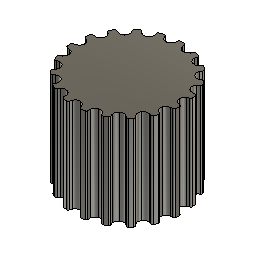
gear_19z (Autodesk Fusion 360 design; units mm, degrees)
Autodesk Fusion 360 part; units mm, degrees
sketch "Sketch1" plane through (0, 0, 0) normal (0, 0, 1) x (1, 0, 0) in component "gt2 pulley"
  circle A0 centre (0, 0) radius 6.0479 construction
  circle A1 centre (0, 0) radius 5.0439 construction
  line L0 (0, 0) -> (0, 6.0479) construction
  line L1 (0, 0) -> (0.9954, 5.9654) construction
  line L2 (0, 0) -> (1.4117, 5.8808) construction
  circle A2 centre (0, 0) radius 5.7939 construction
  arc A3 (0.3524, 5.6394) -> (0.3842, 5.3837) centre (1.3524, 5.6338) ccw
  circle A4 centre (0, 0) radius 5.6439 construction
  arc A5 (0.2077, 5.7902) -> (0, 5.7939) centre (0, 0) ccw
  arc A6 (0.3524, 5.6394) -> (0.2077, 5.7902) centre (0.2024, 5.6403) ccw
  arc A7 (0.3842, 5.3837) -> (0.8302, 4.9751) centre (0.9215, 5.5225) ccw
  arc A8 (0, 5.7939) -> (-0.2077, 5.7902) centre (0, 0) ccw
  arc A9 (-0.2077, 5.7902) -> (-0.3524, 5.6394) centre (-0.2024, 5.6403) ccw
  arc A10 (-0.3842, 5.3837) -> (-0.3524, 5.6394) centre (-1.3524, 5.6338) ccw
  arc A11 (-0.8302, 4.9751) -> (-0.3842, 5.3837) centre (-0.9215, 5.5225) ccw
  arc A12 (0.8302, 4.9751) -> (-0.8302, 4.9751) centre (0, 0) ccw
  point P0 (1.3524, 5.6338)
  point P1 (0, 5.7939)
  dimension "d18" = 12.0958
  dimension "d19" = 9.474
  dimension "d22" = 1.004
  dimension "d24" = 0.75
  dimension "d26" = 1
  dimension "d27" = 0.15
  dimension "d28" = 0.15
  dimension "d47" = 0.555
  dimension "d52" = 3.812
  constraint coincident A0.centre A1.centre
  constraint coincident A0 L0.end
  constraint vertical L0
  constraint coincident A0 L1.end
  constraint coincident A0 L2.end
  constraint concentric A1 A2
  constraint coincident A1 A7.end
  constraint coincident L1 A7.end
  constraint coincident A2 P0
  constraint coincident L2 P0
  constraint coincident P0 A3.centre
  constraint coincident A2 P1
  constraint coincident L0 P1
  constraint concentric A2 A4
  constraint coincident P1 A5.end
  constraint coincident A4 A6.centre
  constraint coincident A3.start A6.start
  constraint tangent A3 A6
  constraint tangent A3 A7
  constraint symmetric L0 A7.end A11.start
  constraint symmetric L0 A3.start A9.end
  constraint symmetric L0 A3.end A10.start
  constraint symmetric L0 A3 A10
  constraint symmetric L0 A5.start A8.end
  constraint symmetric L0 P1 A5.end
  constraint symmetric L0 A5 A8
  constraint symmetric L0 A6 A9
  constraint symmetric L0 A7 A11
  constraint coincident A1 A11.start
  constraint tangent A1 A7
  constraint coincident L1 A7.centre
  measures "d18" diameter of A0
  measures "d19" angle of L0 L1
  measures "d22" distance of A0 A1
  measures "d24" distance of A1 A2
  measures "d26" radius of A3
  measures "d27" distance of A2 A4
  measures "d28" radius of A6
  measures "d47" radius of A7
extrude "Extrude1" add sketch "Sketch1" along normal blind 10 makes body 1
pattern_circular "C-Pattern1" count 19 over 360 about axis through (0, 0, 1.75) along (0, 0, 1) of bodies 1 makes body 2 at (-1.7251, 4.7397, 6.6667) makes body 3 at (-2.562, 4.3448, 3.3333) makes body 4 at (-3.8339, 3.2775, 3.3333) makes body 5 at (-4.9825, 0.7845, 6.6667) makes body 6 at (-5.0386, 0.2316, 3.3333) makes body 7 at (-4.8408, -1.417, 3.3333) makes body 8 at (-4.1184, -2.912, 3.3333) makes body 9 at (-2.9497, -4.0915, 3.3333) makes body 10 at (-1.4614, -4.8275, 3.3333) makes body 11 at (0.1853, -5.0405, 3.3333) makes body 12 at (1.8119, -4.7072, 3.3333) makes body 13 at (3.2421, -3.8638, 3.3333) makes body 14 at (4.6555, -1.9409, 6.6667) makes body 15 at (4.9317, -1.0577, 3.3333) makes body 16 at (5.008, 0.6009, 3.3333) makes body 17 at (3.9517, 3.1344, 6.6667) makes body 18 at (3.0244, 4.0366, 6.6667) makes body 19 at (1.1932, 4.9007, 6.6667)
sketch "Sketch2" plane through (0, 0, 10) normal (0, 0, 1) x (-1, 0, 0)
  arc A0 (-2.1644, -5.2194) -> (-2.0765, -5.409) centre (-2.0228, -5.2689) ccw
  arc A1 (-2.0765, -5.409) -> (-1.6836, -5.5439) centre (0, 0) ccw
  arc A2 (-1.6836, -5.5439) -> (-1.4978, -5.4483) centre (-1.6399, -5.4004) ccw
  arc A3 (-1.3847, -5.2167) -> (-1.4978, -5.4483) centre (-0.5502, -5.7677) ccw
  arc A4 (-0.8302, -4.9751) -> (-1.3847, -5.2167) centre (-0.9215, -5.5225) ccw
  arc A5 (-2.4006, -4.436) -> (-0.8302, -4.9751) centre (0, 0) ccw
  arc A6 (-2.1115, -4.9672) -> (-2.4006, -4.436) centre (-2.6648, -4.9241) ccw
  arc A7 (-2.1644, -5.2194) -> (-2.1115, -4.9672) centre (-3.1084, -4.8895) ccw
  circle A8 centre (0, 0) radius 5.0439
  constraint concentric A1 A8
  constraint coincident A5.start A8
extrude "Extrude2" add sketch "Sketch2" against normal blind 10 contours A5 A8 bodies 1 2 3 4 5 6 7 8 9 10 11 12 13 14 15 16 17 18 19
extrude "Extrude4" [suppressed] in component "gt2 pulley"
pattern_circular "C-Pattern7" [suppressed] in component "gt2 pulley"
extrude "Extrude3" [suppressed] in component "gt2 pulley"
pattern_circular "C-Pattern6" [suppressed] in component "gt2 pulley"
extrude "Extrude2'" [suppressed] in component "gt2 pulley"
pattern_circular "C-Pattern5" [suppressed] in component "gt2 pulley"
extrude "Extrude1'" [suppressed] in component "gt2 pulley"
pattern_circular "C-Pattern4" [suppressed] in component "gt2 pulley"
pattern_circular "C-Pattern3" [suppressed] in component "gt2 pulley"
pattern_circular "C-Pattern2" [suppressed] in component "gt2 pulley"
pattern_circular "C-Pattern1'" [suppressed] in component "gt2 pulley"
copy_body "Body->Comp1" [suppressed] in component "Component"
copy_body "Body->Comp2" [suppressed] in component "Component'"
copy_body "Body->Comp3" [suppressed] in component "Component''"
copy_body "Body->Comp4" [suppressed] in component "Component'''"
copy_body "Body->Comp5" [suppressed] in component "Component''''"
copy_body "Body->Comp6" [suppressed] in component "Component'''''"
copy_body "Body->Comp7" [suppressed] in component "Component''''''"
copy_body "Body->Comp8" [suppressed] in component "Component'''''''"
copy_body "Body->Comp9" [suppressed] in component "Component''''''''"
copy_body "Body->Comp10" [suppressed] in component "Component'''''''''"
copy_body "Body->Comp11" [suppressed] in component "Component''''''''''"
copy_body "Body->Comp12" [suppressed] in component "Component'''''''''''"
copy_body "Body->Comp13" [suppressed] in component "Component''''''''''''"
copy_body "Body->Comp14" [suppressed] in component "Component'''''''''''''"
copy_body "Body->Comp15" [suppressed] in component "Component''''''''''''''"
copy_body "Body->Comp16" [suppressed] in component "Component'''''''''''''''"
copy_body "Body->Comp17" [suppressed] in component "Component''''''''''''''''"
copy_body "Body->Comp18" [suppressed] in component "Component'''''''''''''''''"
copy_body "Body->Comp19" [suppressed] in component "Component''''''''''''''''''"
copy_body "Body->Comp20" [suppressed] in component "Component'''''''''''''''''''"
component "gt2 pulley" placed x (1, 0, 0) y (0, 1, 0) z (0, 0, 1) at (0, 0, 0)
equation "NumTeeth = 19" comment "min 20"
equation "ToothPitch = 2 mm"
equation "PullyDia = NumTeeth * ToothPitch / PI"
equation "ToothAng = ( ( 360 / NumTeeth ) * 1 deg )"
equation "TransOffsetAngle = ToothAng * 0.2"
equation "Sholulder_Radius = 0.15 mm"
equation "Root_Radius = 0.555 mm"
equation "TransRadius = 1 mm"
equation "ToolHeight = 0.75 mm"
equation "PLD = 0.254 mm"
equation "d18 = PullyDia"
equation "d19 = ToothAng / 2"
equation "d22 = PLD + ToolHeight"
equation "d24 = ToolHeight"
equation "d26 = TransRadius"
equation "d27 = Sholulder_Radius"
equation "d31 = NumTeeth"
equation "d33 = NumTeeth"
equation "d35 = NumTeeth"
equation "d37 = NumTeeth"
equation "d41 = NumTeeth"
equation "d45 = NumTeeth"
equation "d47 = Root_Radius"
equation "d50 = NumTeeth"
